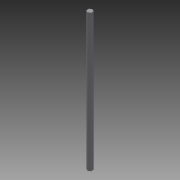
# Autodesk Inventor part: rod3
Saved by Autodesk Inventor 2015 (Build 190159000, 159)
## iProperties
Created: 2016-01-27
Part Number: rod3
Material: Generic
Document SubType Name: Modeling
Designer: 278648
Density: 1 g/cm^3
Appearance: Default
Author: 278648
Autodesk Inventor part; units mm, degrees
ref_plane "YZ Plane" through (0, 0, 0) normal (1, 0, 0) x (0, 1, 0)
ref_plane "XZ Plane" through (0, 0, 0) normal (0, 1, 0) x (-1, 0, 0)
ref_plane "XY Plane" through (0, 0, 0) normal (0, 0, 1) x (1, 0, 0)
sketch "Sketch1" plane through (0, 0, 0) normal (0, 1, 0) x (-1, 0, 0)
  line L0 (0, -7.3323) -> (-6.35, -3.6662)
  line L1 (-6.35, -3.6662) -> (-6.35, 3.6662)
  line L2 (-6.35, 3.6662) -> (0, 7.3323)
  line L3 (0, 7.3323) -> (6.35, 3.6662)
  line L4 (6.35, 3.6662) -> (6.35, -3.6662)
  line L5 (6.35, -3.6662) -> (0, -7.3323)
  point P0 (0, 0)
  point P1 (0, 0)
  dimension "d0" = 12.7
  constraints: 12 end point, 1 coincident, 13 other
  measures "d0" distance between parallel lines of L3 L0
extrude "Extrusion1" add sketch "Sketch1" along normal blind 406.4
body "Solid1"
